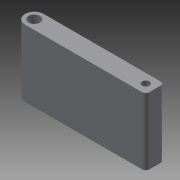
# Autodesk Inventor part: porte
Saved by Autodesk Inventor 2015 (Build 190159000, 159)
## iProperties
Created: 2015-02-17
Part Number: porte
Material: Generic
Document SubType Name: Modeling
Designer: Piotr
Density: 1 g/cm^3
Appearance: Default
Author: Piotr
Autodesk Inventor part; units mm, degrees
ref_plane "YZ Plane" through (0, 0, 0) normal (1, 0, 0) x (0, 1, 0)
ref_plane "XZ Plane" through (0, 0, 0) normal (0, 1, 0) x (-1, 0, 0)
ref_plane "XY Plane" through (0, 0, 0) normal (0, 0, 1) x (1, 0, 0)
sketch "Sketch1" plane through (0, 0, 0) normal (0, 0, 1) x (1, 0, 0)
  line L0 (0, 0) -> (35, 0)
  line L1 (35, 0) -> (35, -5)
  line L2 (35, -5) -> (0, -5)
  line L3 (0, -5) -> (0, 0)
  dimension "d0" = 35
  dimension "d1" = 5
  constraints: 8 end point, 2 parallel, 1 horizontal, 1 perpendicular
  measures "d0" distance of L0.start L0.end
  measures "d1" distance of L2.end L0.start
extrude "Extrusion1" add sketch "Sketch1" along normal blind 18
sketch "Sketch2" plane through (0, 0, 18) normal (0, 0, 1) x (1, 0, 0)
  line L0 (0, 0) -> (0, -5) projected
  line L1 (0, 0) -> (35, 0) projected
  point P0 (2.5, -2.5)
  dimension "d4" = 2.5
  dimension "d5" = 2.5
  measures "d4" distance from line of L0 point (2.5, -2.5)
  measures "d5" distance from line of L1 point (2.5, -2.5)
hole "Hole1" at (2.5, -2.5, 18) direction (0, 0, -1) diameter 3.1 end through all
fillet "Fillet1" radius 1 2 edges at (35, -5, 9) (35, 0, 9)
fillet "Fillet2" radius 2.5 2 edges at (0, -5, 9) (0, 0, 9)
sketch "Sketch3" plane through (0, 0, 18) normal (0, 0, 1) x (1, 0, 0)
  circle A0 centre (2.5, -2.5) radius 1.55 construction
  line L0 (2.5, -5) -> (34, -5) construction
  line L1 (34, 0) -> (2.5, 0) construction
  line L2 (35, -4) -> (35, -1) construction
  point P0 (0, 0)
  point P1 (32.5, -2.5)
  dimension "d15" = 2.5
  dimension "d16" = 2.5
  dimension "d17" = 5
  measures "d15" distance from line of L2 point (32.5, -2.5)
  measures "d16" distance from line of point (32.5, -2.5) L1
  measures "d17" distance between parallel lines of L0 L1
hole "Hole2" at (32.5, -2.5, 18) direction (0, 0, -1) diameter 2 depth 11 tip angle 118
equation "\"d15\" = 0.5 * d17"
equation "\"d16\" = d15"
body "Solid1"
